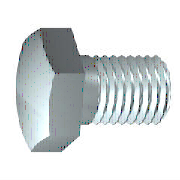
# Autodesk Inventor part: ANSI B18.2.3.5M - M10 x 1,5 x 70
Saved by Autodesk Inventor 2023 (Build 270158000, 158)
## iProperties
Created: 2022-02-04
Part Number: ANSI B18.2.3.5M - M10 x 1,5 x 70
Material: Сталь, мягкая
Description: Болт с шестигранной головкой
Document SubType Name: Modeling
Standard: ANSI B18.2.3.5M
Designer: eliza
Standard Revision: 1979 (R2001)
Standards Organization: ANSI
Language: ru-RU
Size Designation: M10 x 1,5 x 70
Categories: <MemberInstance><Categories><Category DisplayName="Крепежные изделия" InternalName="e4da775c-781d-43d5-af7c-5136215cf5a6" Mnemonic="FSTN"><Category DisplayName="Болты  Винты" InternalName="536e6df0-f778-49ac-b2f2-25c71d2aa0b2" Mnemonic="SCRW"><CategoryParameter DisplayName="Обозначение номинального диаметра" InternalName="03caf894-eafd-4c09-a035-916ac084b87b" Mnemonic="nomdiadesig"/><CategoryParameter DisplayName="Номинальная длина" InternalName="238ecbaf-3e6c-45dd-aa95-4068c8e0fd02" Mnemonic="nomlen"/><CategoryParameter DisplayName="Обозначение резьбы" InternalName="586d5e89-370a-4089-914f-0110033585c7" Mnemonic="thrdesign"/><CategoryParameter DisplayName="Обозначение серии резьб" InternalName="87c5849c-b3a5-4c3e-9c9b-2feecef9be86" Mnemonic="thrserdsgn"/><CategoryParameter DisplayName="Номинальный диаметр" InternalName="8bbe3f8e-44cf-40a9-a251-3a6edc8168d6" Mnemonic="nomdia"/><CategoryParameter DisplayName="Тип резьбы" InternalName="b4bbb7bc-d6aa-4c9f-a9a9-4152b9f6fe49" Mnemonic="thrtype"/><CategoryParameter DisplayName="Шаг резьбы" InternalName="bb82302e-82d8-4176-8fc1-c5d7bb17d5ad" Mnemonic="pitch1"/><CategoryParameter DisplayName="Витков на единицу" InternalName="bdc6e7d2-ffd0-4d9c-a173-16b95ebb912d" Mnemonic="thrperunit1"/><CategoryParameter DisplayName="Класс резьбы" InternalName="ebc0d23b-2cc6-4d2a-b376-d52aae53bab6" Mnemonic="thrclss"/><Category DisplayName="С шестигранной головкой" InternalName="520da9a1-ead7-4898-b571-59b4b339a5c6" Mnemonic="PLSCRW"><CategoryParameter DisplayName="Длина стержня" InternalName="14b808f1-b175-4f80-b2c8-3c2ac1acde4c" Mnemonic="grplen"/><CategoryParameter DisplayName="Ширина по плоскостям" InternalName="1cb53529-b7fd-49c5-a5c5-85a22d509c9e" Mnemonic="waflat"/><CategoryParameter DisplayName="Высота головки" InternalName="3a45ce7b-b38d-4f77-aad7-a2328eea5aef" Mnemonic="headh"/><CategoryParameter DisplayName="Длина резьбы" InternalName="50b9771a-9fb7-48bc-803b-80099da79f2d" Mnemonic="thrlen"/><CategoryParameter DisplayName="Ширина по углам" InternalName="a21dc55e-7dbc-4faf-83dd-c7c1bfd07428" Mnemonic="wacor"/><CategoryParameter DisplayName="Диаметр стержня" InternalName="bad16e07-a90c-44cc-a6af-8a6b56171876" Mnemonic="grpdia"/><CategoryParameter DisplayName="Диаметр контактной поверхности" InternalName="cc3b219b-8087-4820-96e9-69a08f47c1a6" Mnemonic="conardia"/></Category></Category></Category><Category DisplayName="ТипДанных" InternalName="23b78d0f-2648-40c6-8793-ca6db495c9e8" Mnemonic="DATATYPE"><CategoryParameter DisplayName="ОтображаемоеИмя" InternalName="05415f3d-3907-474b-a020-eb9d644f4cf3" Mnemonic="DISPLAYNAME"/><CategoryParameter DisplayName="Стандарт" InternalName="0c0a119c-1e12-4c84-803f-101930972f5e" Mnemonic="STANDARD"/><CategoryParameter DisplayName="Наименование" InternalName="13903e3d-64b1-4950-80da-f627842ea37f" Mnemonic="DESCRIPTION"/><CategoryParameter DisplayName="Обозначение" InternalName="2675968c-4ce5-49e0-a4f5-552d29089031" Mnemonic="DESIGNATION"/><CategoryParameter DisplayName="Строка по умолчанию" InternalName="2af9ec52-faaa-4026-b378-f9fa4afca842" Mnemonic="DEFAULTROW"/><CategoryParameter DisplayName="Имя папки" InternalName="3f06958e-8713-4116-9be7-ed6184ecc97b" Mnemonic="FOLDERNAME"/><CategoryParameter DisplayName="Указатель редакций" InternalName="45a75005-10b1-4dfc-8d6d-dfe629f0b93c" Mnemonic="REVISIONGUID"/><CategoryParameter DisplayName="ИмяФайла" InternalName="8b46a4cc-9585-4fed-90c3-899f57e09a73" Mnemonic="FILENAME"/><CategoryParameter DisplayName="ОргСтанд" InternalName="8f5914e1-4693-403f-8ab5-d37768198c9d" Mnemonic="STDSORG"/><CategoryParameter DisplayName="Версия семейства" InternalName="914462f6-6e19-4b14-ba84-155b9680b1d0" Mnemonic="FAMILYREVISION"/><CategoryParameter DisplayName="Редакция стандарта" InternalName="91d5a463-65c2-4fde-b823-3b7fea5e8e17" Mnemonic="STANDARDREVISION"/><CategoryParameter DisplayName="редакция элемента" InternalName="a65d44b9-392f-4f4f-857b-e4b3d54996fe" Mnemonic="MEMBERREVISION"/><CategoryParameter DisplayName="ФорматКлипа" InternalName="bc51e27b-3422-4e78-93ef-cec197ddf230" Mnemonic="CLIPFORMAT"/><CategoryParameter DisplayName="Изготовитель" InternalName="cd6c7a72-a28a-4e50-99a9-2c7f4e13e5ad" Mnemonic="MANUFACTURER"/><CategoryParameter DisplayName="ВнутреннееИмя" InternalName="cf1d0246-76d9-4b4a-8305-fa0409afb5c1" Mnemonic="INTERNALNAME"/><CategoryParameter DisplayName="Метрическая" InternalName="e2385c5b-1ea4-4823-96a8-8de651266ec3" Mnemonic="ISMETRIC"/><Category DisplayName="Деталь" InternalName="c0e0b642-3bcb-4cc8-9e80-f96d35c4afa4" Mnemonic="PART"><CategoryParameter DisplayName="Номер детали" InternalName="016b6077-bfbe-49bd-92c9-d8d59c39c941" Mnemonic="PARTNUMBER"/><CategoryParameter DisplayName="Инвентарный номер" InternalName="4dba7c1c-e26c-444e-836c-b08b433409a8" Mnemonic="STOCKNUMBER"/><CategoryParameter DisplayName="Ключ материала" InternalName="5c9a8adb-dd2b-4535-b97f-0a94a95fe41f" Mnemonic="MATERIALKEY"/><CategoryParameter DisplayName="Материал" InternalName="818a152a-d3c3-49ca-80ee-df7d91421b8e" Mnemonic="MATERIAL"/></Category></Category><Category DisplayName="СтараяКарта" InternalName="cd87c42b-3e48-431e-b5c0-1cbeb14dfe77" Mnemonic="LEGACYMAP"><CategoryParameter DisplayName="уникальное обозначение элемента DA" InternalName="0918ad47-427f-4fed-ae26-24c81c58f590" Mnemonic="DACOOKIE"/><CategoryParameter DisplayName="Объединить код 11" InternalName="0ee8fb18-e2ed-4f39-96f6-1f4b5f50aa71" Mnemonic="MERGE11"/><CategoryParameter DisplayName="уникальное обозначение элемента CC" InternalName="5193edd4-b2b0-4ab4-9d54-de900eee34e0" Mnemonic="CCCOOKIE"/><CategoryParameter DisplayName="Разделить код" InternalName="72b5c83c-be7f-45c4-ae51-9160ea6deb26" Mnemonic="SPLIT"/><CategoryParameter DisplayName="КодУчастника" InternalName="8e5e0294-fc51-4c8f-b3d7-003dc5ed94f6" Mnemonic="MEMBERID"/><CategoryParameter DisplayName="ИмяКаталога" InternalName="d99d1e27-aa94-4de2-af4c-c348882a6f4f" Mnemonic="CATALOGNAME"/><CategoryParameter DisplayName="НомерСемейства" InternalName="e705e1f4-09cb-413e-91f9-551b4188271e" Mnemonic="FAMILYNUMBER"/></Category></Categories><FamilyTemplate Id="si00021"><FamilyTemplateParameters><FamilyTemplateParameter ObjectType="kUserParameterObject" ValueType="xs:double" Id="1" ObjectReferenceKey="GUL"/><FamilyTemplateParameter ObjectType="kUserParameterObject" ValueType="xs:double" Id="2" ObjectReferenceKey="SPD"/><FamilyTemplateParameter ObjectType="kUserParameterObject" ValueType="xs:double" Id="3" ObjectReferenceKey="GD"/><FamilyTemplateParameter ObjectType="kUserParameterObject" ValueType="xs:double" Id="4" ObjectReferenceKey="TPU"/><FamilyTemplateParameter ObjectType="kUserParameterObject" ValueType="xs:double" Id="5" ObjectReferenceKey="GD1"/><FamilyTemplateParameter ObjectType="kUserParameterObject" ValueType="xs:double" Id="6" ObjectReferenceKey="GEL"/><FamilyTemplateParameter ObjectType="kUserParameterObject" ValueType="xs:double" Id="7" ObjectReferenceKey="SW"/><FamilyTemplateParameter ObjectType="kUserParameterObject" ValueType="xs:double" Id="8" ObjectReferenceKey="THREADDIA"/><FamilyTemplateParameter ObjectType="kUserParameterObject" ValueType="xs:double" Id="9" ObjectReferenceKey="ANG1"/><FamilyTemplateParameter ObjectType="kUserParameterObject" ValueType="xs:double" Id="10" ObjectReferenceKey="TOA"/><FamilyTemplateParameter ObjectType="kUserParameterObject" ValueType="xs:double" Id="11" ObjectReferenceKey="BDM"/><FamilyTemplateParameter ObjectType="kUserParameterObject" ValueType="xs:double" Id="12" ObjectReferenceKey="NLG"/><FamilyTemplateParameter ObjectType="kUserParameterObject" ValueType="xs:double" Id="13" ObjectReferenceKey="KOH"/><FamilyTemplateParameter ObjectType="kUserParameterObject" ValueType="xs:double" Id="14" ObjectReferenceKey="PTC"/><FamilyTemplateParameter ObjectType="kUserParameterObject" ValueType="xs:double" Id="15" ObjectReferenceKey="KOH1"/><FamilyTemplateParameter ObjectType="kUserParameterObject" ValueType="xs:double" Id="16" ObjectReferenceKey="NND"/><FamilyTemplateParameter ObjectType="kUserParameterObject" ValueType="xs:double" Id="17" ObjectReferenceKey="RR1"/><FamilyTemplateParameter ObjectType="kUserParameterObject" ValueType="xs:double" Id="18" ObjectReferenceKey="SW0"/><FamilyTemplateParameter ObjectType="kUserParameterObject" ValueType="xs:double" Id="19" ObjectReferenceKey="GAL"/><FamilyTemplateParameter ObjectType="kUserParameterObject" ValueType="xs:double" Id="20" ObjectReferenceKey="SD"/><FamilyTemplateParameter ObjectType="kUserParameterObject" ValueType="xs:double" Id="21" ObjectReferenceKey="SD2"/><FamilyTemplateParameter ObjectType="kUserParameterObject" ValueType="xs:double" Id="22" ObjectReferenceKey="E0"/><FamilyTemplateParameter ObjectType="kPropertyObject" ValueType="xs:string" Id="100" ObjectReferenceKey="{32853F0F-3444-11d1-9E93-0060B03C1CA6}" SubObjectId="52"/><FamilyTemplateParameter ObjectType="kPropertyObject" ValueType="xs:string" Id="105" ObjectReferenceKey="{32853F0F-3444-11d1-9E93-0060B03C1CA6}" SubObjectId="5"/><FamilyTemplateParameter ObjectType="kPartComponentDefinitionObject" ValueType="xs:string" Id="110" SubObjectId="Material"/><FamilyTemplateParameter ObjectType="kThreadFeatureObject" ValueType="xs:structure" Id="300" ObjectReferenceKey="100200001000000049150000000000008000000000000000" SubObjectId="ThreadInfo"><FamilyTemplateParameter ObjectType="" ValueType="xs:string" Id="301" SubObjectId="ThreadDesignation"/><FamilyTemplateParameter ObjectType="" ValueType="xs:string" Id="302" SubObjectId="ThreadType"/><FamilyTemplateParameter ObjectType="" ValueType="xs:string" Id="303" SubObjectId="ThreadClass"/></FamilyTemplateParameter></FamilyTemplateParameters></FamilyTemplate><CategoryParameterMap><ParamToTemplateMap><ParamToTemplate CategoryParameter="//CategoryParameter[@InternalName='05415f3d-3907-474b-a020-eb9d644f4cf3']" ConstantValue="Hex Bolt - Metric"/><ParamToTemplate CategoryParameter="//CategoryParameter[@InternalName='cf1d0246-76d9-4b4a-8305-fa0409afb5c1']" ConstantValue="b58bfb06-034c-416d-a616-37d628731a36"/><ParamToTemplate CategoryParameter="//CategoryParameter[@InternalName='3f06958e-8713-4116-9be7-ed6184ecc97b']" ConstantValue="ANSI B18.2.3.5M"/><ParamToTemplate CategoryParameter="//CategoryParameter[@InternalName='914462f6-6e19-4b14-ba84-155b9680b1d0']" ConstantValue="10"/><ParamToTemplate CategoryParameter="//CategoryParameter[@InternalName='bc51e27b-3422-4e78-93ef-cec197ddf230']" ConstantValue="CF_INVENTOR.STDPARTS"/><ParamToTemplate CategoryParameter="//CategoryParameter[@InternalName='e2385c5b-1ea4-4823-96a8-8de651266ec3']" ConstantValue="true"/><ParamToTemplate CategoryParameter="//CategoryParameter[@InternalName='13903e3d-64b1-4950-80da-f627842ea37f']" ConstantValue="Hex Bolt"/><ParamToTemplate CategoryParameter="//CategoryParameter[@InternalName='8f5914e1-4693-403f-8ab5-d37768198c9d']" ConstantValue="ANSI"/><ParamToTemplate CategoryParameter="//CategoryParameter[@InternalName='0c0a119c-1e12-4c84-803f-101930972f5e']" ConstantValue="ANSI B18.2.3.5M"/><ParamToTemplate CategoryParameter="//CategoryParameter[@InternalName='cd6c7a72-a28a-4e50-99a9-2c7f4e13e5ad']" TemplateParameter="104"/><ParamToTemplate CategoryParameter="//CategoryParameter[@InternalName='91d5a463-65c2-4fde-b823-3b7fea5e8e17']" ConstantValue="1979 (R2001)"/><ParamToTemplate CategoryParameter="//CategoryParameter[@InternalName='45a75005-10b1-4dfc-8d6d-dfe629f0b93c']" ConstantValue="e8be81b6-7891-4da8-bbc6-1513e23f7eaf"/><ParamToTemplate CategoryParameter="//CategoryParameter[@InternalName='2af9ec52-faaa-4026-b378-f9fa4afca842']" ConstantValue="10"/><ParamToTemplate CategoryParameter="//CategoryParameter[@InternalName='d99d1e27-aa94-4de2-af4c-c348882a6f4f']" ConstantValue="ANSI"/><ParamToTemplate CategoryParameter="//CategoryParameter[@InternalName='e705e1f4-09cb-413e-91f9-551b4188271e']" ConstantValue="78"/><ParamToTemplate CategoryParameter="//CategoryParameter[@InternalName='8b46a4cc-9585-4fed-90c3-899f57e09a73']" ConstantValue="ANSI B18.2.3.5M - M10 x 1,5 x 70"/><ParamToTemplate CategoryParameter="//CategoryParameter[@InternalName='a65d44b9-392f-4f4f-857b-e4b3d54996fe']" ConstantValue="8AB0CEC1-37A4-4226-8EEC-C9487C5EECA2"/><ParamToTemplate CategoryParameter="//CategoryParameter[@InternalName='14b808f1-b175-4f80-b2c8-3c2ac1acde4c']" ConstantValue="44"/><ParamToTemplate CategoryParameter="//CategoryParameter[@InternalName='ebc0d23b-2cc6-4d2a-b376-d52aae53bab6']" ConstantValue="6g"/><ParamToTemplate CategoryParameter="//CategoryParameter[@InternalName='03caf894-eafd-4c09-a035-916ac084b87b']" ConstantValue="M10"/><ParamToTemplate CategoryParameter="//CategoryParameter[@InternalName='b4bbb7bc-d6aa-4c9f-a9a9-4152b9f6fe49']" ConstantValue="ISO Metric profile"/><ParamToTemplate CategoryParameter="//CategoryParameter[@InternalName='8e5e0294-fc51-4c8f-b3d7-003dc5ed94f6']" ConstantValue="510"/><ParamToTemplate CategoryParameter="//CategoryParameter[@InternalName='bad16e07-a90c-44cc-a6af-8a6b56171876']" TemplateParameter="11"/><ParamToTemplate CategoryParameter="//CategoryParameter[@InternalName='2675968c-4ce5-49e0-a4f5-552d29089031']" TemplateParameter="100"/><ParamToTemplate CategoryParameter="//CategoryParameter[@InternalName='a21dc55e-7dbc-4faf-83dd-c7c1bfd07428']" TemplateParameter="22"/><ParamToTemplate CategoryParameter="//CategoryParameter[@InternalName='50b9771a-9fb7-48bc-803b-80099da79f2d']" TemplateParameter="6"/><ParamToTemplate CategoryParameter="//CategoryParameter[@InternalName='3a45ce7b-b38d-4f77-aad7-a2328eea5aef']" TemplateParameter="13"/><ParamToTemplate CategoryParameter="//CategoryParameter[@InternalName='818a152a-d3c3-49ca-80ee-df7d91421b8e']" TemplateParameter="110"/><ParamToTemplate CategoryParameter="//CategoryParameter[@InternalName='238ecbaf-3e6c-45dd-aa95-4068c8e0fd02']" TemplateParameter="12"/><ParamToTemplate CategoryParameter="//CategoryParameter[@InternalName='8bbe3f8e-44cf-40a9-a251-3a6edc8168d6']" TemplateParameter="16"/><ParamToTemplate CategoryParameter="//CategoryParameter[@InternalName='016b6077-bfbe-49bd-92c9-d8d59c39c941']" TemplateParameter="105"/><ParamToTemplate CategoryParameter="//CategoryParameter[@InternalName='bb82302e-82d8-4176-8fc1-c5d7bb17d5ad']" TemplateParameter="14"/><ParamToTemplate CategoryParameter="//CategoryParameter[@InternalName='586d5e89-370a-4089-914f-0110033585c7']" TemplateParameter="301"/><ParamToTemplate CategoryParameter="//CategoryParameter[@InternalName='bdc6e7d2-ffd0-4d9c-a173-16b95ebb912d']" TemplateParameter="4"/></ParamToTemplateMap></CategoryParameterMap></MemberInstance>
Density: 7.85 g/cm^3
Appearance: С умеренной полировкой
IsCustomPart: 0
Author: eliza
Autodesk Inventor part; units mm, degrees
ref_plane "YZ Plane" through (0, 0, 0) normal (1, 0, 0) x (0, 1, 0)
ref_plane "XZ Plane" through (0, 0, 0) normal (0, 1, 0) x (-1, 0, 0)
sketch "Эскиз1" plane through (0, 0, 0) normal (0, 0, 1) x (1, 0, 0)
  line L0 (0, 5) -> (70, 5)
  line L1 (70, 5) -> (70, 0)
  line L2 (70, 0) -> (0, 0)
  line L3 (-14, 0) -> (84, 0) projected
  line L4 (0, -1) -> (0, 6) projected
  line L5 (0, 5) -> (0, 0)
  dimension "d2" = 10
  dimension "d59" = 70
  constraints: 8 end point, 3 point on line, 1 collinear
  measures "d2" diameter of L0 L2
  measures "d59" distance between parallel lines of L1 L4
revolve "Базовый элемент" add sketch "Эскиз1" angle 360 about axis through (70, 0, 0) along (-1, 0, 0)
sketch "Эскиз2" plane through (0, 0, 0) normal (-1, 0, 0) x (0, 0, 1)
  line L0 (0, 9.2376) -> (8, 4.6188)
  line L1 (8, 4.6188) -> (8, -4.6188)
  line L2 (8, -4.6188) -> (0, -9.2376)
  line L3 (0, -9.2376) -> (-8, -4.6188)
  line L4 (-8, -4.6188) -> (-8, 4.6188)
  line L5 (-8, 4.6188) -> (0, 9.2376)
  line L6 (-11.2, 0) -> (11.2, 0) projected
  line L7 (0, 12.9326) -> (0, -12.9326) projected
  point P0 (0, 0)
  point P1 (0, 0)
  dimension "d11" = 16
  constraints: 12 end point, 2 midpoint, 1 coincident, 1 vertical, 11 other
  measures "d11" distance between parallel lines of L4 L1
extrude "С головкой" add sketch "Эскиз2" along normal blind 6.85
sketch "Эскиз4" plane through (0, 0, 0) normal (0, 0, 1) x (1, 0, 0)
  line L0 (-5.9262, 9.6) -> (-6.85, 8)
  line L1 (-1.1, 0) -> (-0.234, 0)
  line L2 (-8.1732, 0) -> (1.0892, 0) projected
  line L3 (-6.85, 9.6) -> (-5.9262, 9.6)
  line L4 (-6.85, 8) -> (-6.85, 9.6)
  line L5 (0, 11.52) -> (0, -1.92) projected
  dimension "d65" = 16
  dimension "d67" = 30
  dimension "d68" = 19.2
  dimension "d69" = 6.85
  constraints: 8 end point, 1 parallel, 1 perpendicular, 1 point on line
  measures "d65" diameter of L0.end L1
  measures "d67" angle of L0 L4
  measures "d68" diameter of L3 L1
  measures "d69" distance between parallel lines of L4 L5
revolve "Фаска1" cut sketch "Эскиз4" angle 360 about axis through (-1.1, 0, 0) along (1, 0, 0)
thread "Резьба" size "M10x1.5" class "6g" standard "ISO Metric profile" length 26
chamfer "Фаска2" distance 0.9202 distance2 0.9203 1 edges at (70, -5, 0) measured on face at (70, -2.0394, -1.2014)
fillet "Fillet" radius 0.4 1 edges at (0, -5, 0)
ref_plane "Work Plane1" through (1.525, 0, 0) normal (0, 0, 1) x (1, 0, 0)
equation "\"d2\" = GD"
equation "\"d59\" = NLG"
equation "\"d11\" = SW"
equation "\"d3\" = KOH"
equation "\"d71\" = RR1"
equation "\"d15\" = GEL"
equation "\"d6\" = -0.5 * SPD + 0.5 * GD"
equation "\"d65\" = SW"
equation "\"d67\" = ANG1"
equation "\"d68\" = 1.2 * SW"
equation "\"d69\" = KOH"
equation "\"NLG\" = 70"
equation "\"GD\" = NND"
equation "\"KOH\" = 6.85"
equation "\"GEL\" = 26"
equation "\"SW\" = 16"
equation "\"SW0\" = SW"
equation "\"SPD\" = NND - 1.2269 * PTC"
equation "\"SD\" = 0"
equation "\"ANG1\" = 30deg"
equation "\"GAL\" = 0.61345 * PTC"
equation "\"GUL\" = 0.61345 * PTC"
equation "\"RR\" = 0.1"
equation "\"RR1\" = 0.4"
equation "\"GD1\" = THREADDIA - 1.2269 * PTC"
equation "\"TOA\" = 30deg"
equation "\"PTC\" = 1.5"
equation "\"KOH1\" = 4.5"
equation "\"E0\" = 1.155 * SW"
equation "\"NND\" = 10"
equation "\"THREADDIA\" = 10"
body "Solid1"
